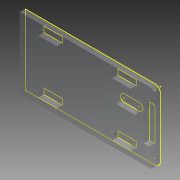
# Autodesk Inventor part: motor mount top
Saved by Autodesk Inventor 2015 (Build 190159000, 159)
## iProperties
Created: 2015-10-17
Part Number: motor mount top
Material: Polycarbonate, Clear
Document SubType Name: Modeling
Designer: Brian
Density: 1.2 g/cm^3
Appearance: Polycarbonate - Clear
Mass: 9.18565 g
Surface Area: 62.8512 cm^2
Volume: 7.65471 cm^3
Author: Brian
Autodesk Inventor part; units mm, degrees
ref_plane "YZ Plane" through (0, 0, 0) normal (1, 0, 0) x (0, 1, 0)
ref_plane "XZ Plane" through (0, 0, 0) normal (0, 1, 0) x (-1, 0, 0)
ref_plane "XY Plane" through (0, 0, 0) normal (0, 0, 1) x (1, 0, 0)
sketch "Sketch1" plane through (0, 0, 0) normal (0, 1, 0) x (-1, 0, 0)
  line L0 (0, 0) -> (73, 0)
  line L1 (73, 0) -> (73, -38)
  line L2 (73, -38) -> (0, -38)
  line L3 (0, -38) -> (0, 0)
  line L4 (13, -35) -> (23, -35)
  line L5 (23, -35) -> (23, -32)
  line L6 (23, -32) -> (13, -32)
  line L7 (13, -32) -> (13, -35)
  line L8 (3, -28) -> (6, -28)
  line L9 (6, -28) -> (6, -10)
  line L10 (6, -10) -> (3, -10)
  line L11 (3, -10) -> (3, -28)
  line L12 (13, -6) -> (23, -6)
  line L13 (23, -6) -> (23, -3)
  line L14 (23, -3) -> (13, -3)
  line L15 (13, -3) -> (13, -6)
  line L16 (63, -3) -> (53, -3)
  line L17 (53, -3) -> (53, -6)
  line L18 (53, -6) -> (63, -6)
  line L19 (63, -6) -> (63, -3)
  line L20 (63, -32) -> (53, -32)
  line L21 (53, -32) -> (53, -35)
  line L22 (53, -35) -> (63, -35)
  line L23 (63, -35) -> (63, -32)
  point P0 (3, -19)
  point P1 (0, -19)
  dimension "d0" = 73
  dimension "d1" = 38
  dimension "d3" = 3
  dimension "d4" = 3
  dimension "d5" = 3
  dimension "d6" = 10
  dimension "d7" = 10
  dimension "d8" = 18
  dimension "d9" = 32
  dimension "d10" = 3
  dimension "d11" = 3
  dimension "d12" = 3
  dimension "d13" = 10
  dimension "d14" = 13
  constraints: 48 end point, 12 parallel, 6 horizontal, 6 perpendicular, 5 point on line, 3 collinear, 2 midpoint, 1 horizontal alignment
  measures "d0" distance of L0.start L0.end
  measures "d1" distance of L2.end L0.start
  measures "d3" distance between parallel lines of L3 L11
  measures "d4" distance of L14.end L12.start
  measures "d5" distance of L22.end L20.start
  measures "d6" distance of L4.start L4.end
  measures "d7" distance of L21.end L22.end
  measures "d8" distance of L10.end L8.start
  measures "d9" distance between parallel lines of L14 L4
  measures "d10" distance between parallel lines of L2 L4
  measures "d11" distance between parallel lines of L0 L14
  measures "d12" distance of L8.start L8.end
  measures "d13" distance between parallel lines of L1 L23
  measures "d14" distance between parallel lines of L3 L15
extrude "Extrusion1" add sketch "Sketch1" along normal blind 3
fillet "Fillet1" radius 3 2 edges at (0, 1.5, 0) (0, 1.5, -38)
sketch "Sketch2" plane through (0, 0, 0) normal (0, -1, 0) x (1, 0, 0)
  line L0 (-3, -10) -> (-3, -28) projected
  line L1 (-3, -28) -> (-6, -28) projected
  line L2 (-6, -28) -> (-6, -10) projected
  line L3 (-6, -10) -> (-3, -10) projected
  line L4 (-63, -35) -> (-63, -32) projected
  line L5 (-63, -32) -> (-53, -32) projected
  line L6 (-53, -32) -> (-53, -35) projected
  line L7 (-53, -35) -> (-63, -35) projected
  line L8 (-63, -6) -> (-63, -3) projected
  line L9 (-63, -3) -> (-53, -3) projected
  line L10 (-53, -3) -> (-53, -6) projected
  line L11 (-53, -6) -> (-63, -6) projected
  line L12 (-13, -3) -> (-13, -6) projected
  line L13 (-13, -6) -> (-23, -6) projected
  line L14 (-23, -6) -> (-23, -3) projected
  line L15 (-23, -3) -> (-13, -3) projected
  line L16 (-13, -32) -> (-13, -35) projected
  line L17 (-13, -35) -> (-23, -35) projected
  line L18 (-23, -35) -> (-23, -32) projected
  line L19 (-23, -32) -> (-13, -32) projected
  arc A0 (-3, -38) -> (0, -35) centre (-3, -35) ccw projected
  line L20 (0, -35) -> (0, -3) projected
  arc A1 (0, -3) -> (-3, 0) centre (-3, -3) ccw projected
  line L21 (-3, 0) -> (-73, 0) projected
  line L22 (-73, 0) -> (-73, -38) projected
  line L23 (-73, -38) -> (-3, -38) projected
  line L24 (-9.5, -15) -> (-21.5, -15) construction
  line L25 (-11.5, -17) -> (-19.5, -17)
  line L26 (-19.5, -13) -> (-11.5, -13)
  arc A2 (-11.5, -17) -> (-11.5, -13) centre (-11.5, -15) ccw
  arc A3 (-19.5, -13) -> (-19.5, -17) centre (-19.5, -15) ccw
  line L27 (-73, 0) -> (-73, -38) projected
  point P0 (0, 0)
  point P1 (-73, -19)
  point P2 (-15.5, -15)
  point P3 (-73, -19)
  dimension "d21" = 2
  dimension "d22" = 8
  dimension "d23" = 11.5
  dimension "d26" = 15
  constraints: 8 end point, 7 point on circle, 4 tangent, 3 midpoint, 2 centre point, 2 point on line, 1 horizontal, 1 parallel
  measures "d21" radius of A2
  measures "d22" distance of L26.start L26.end
  measures "d23" distance from line of L20 A2.centre
  measures "d26" distance between parallel lines of L21 L24
extrude "Extrusion2" cut sketch "Sketch2" against normal blind 3 contours L25 A3 L26 A2
sketch "Sketch3" plane through (0, 3, 0) normal (0, 1, 0) x (1, 0, 0)
  arc A0 (-11.5, 13) -> (-11.5, 17) centre (-11.5, 15) ccw projected
  line L0 (-11.5, 13) -> (-19.5, 13) projected
  arc A1 (-19.5, 17) -> (-19.5, 13) centre (-19.5, 15) ccw projected
  line L1 (-19.5, 17) -> (-11.5, 17) projected
  arc A2 (0, 35) -> (-3, 38) centre (-3, 35) ccw projected
  line L2 (-3, 38) -> (-73, 38) projected
  line L3 (-73, 38) -> (-73, 0) projected
  line L4 (-73, 0) -> (-3, 0) projected
  arc A3 (-3, 0) -> (0, 3) centre (-3, 3) ccw projected
  line L5 (0, 3) -> (0, 35) projected
  line L6 (-3, 28) -> (-3, 10) projected
  line L7 (-3, 10) -> (-6, 10) projected
  line L8 (-6, 10) -> (-6, 28) projected
  line L9 (-6, 28) -> (-3, 28) projected
  line L10 (-63, 32) -> (-63, 35) projected
  line L11 (-63, 35) -> (-53, 35) projected
  line L12 (-53, 35) -> (-53, 32) projected
  line L13 (-53, 32) -> (-63, 32) projected
  line L14 (-63, 3) -> (-63, 6) projected
  line L15 (-63, 6) -> (-53, 6) projected
  line L16 (-53, 6) -> (-53, 3) projected
  line L17 (-53, 3) -> (-63, 3) projected
  line L18 (-13, 6) -> (-13, 3) projected
  line L19 (-13, 3) -> (-23, 3) projected
  line L20 (-23, 3) -> (-23, 6) projected
  line L21 (-23, 6) -> (-13, 6) projected
  line L22 (-13, 35) -> (-13, 32) projected
  line L23 (-13, 32) -> (-23, 32) projected
  line L24 (-23, 32) -> (-23, 35) projected
  line L25 (-23, 35) -> (-13, 35) projected
  point P0 (0, 0)
equation "\"d5\" = d4"
equation "\"d10\" = d11"
body "Solid1"
